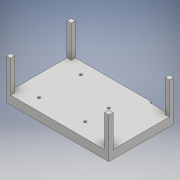
# Autodesk Inventor part: Back Plate test02
Saved by Autodesk Inventor 2018 (Build 220112000, 112)
## iProperties
Created: 2022-01-10
Part Number: Back Plate test02
Material: Generic
Document SubType Name: Modeling
Designer: Stewart Alexander
Density: 1 g/cm^3
Appearance: Default
Author: Stewart Alexander
Autodesk Inventor part; units mm, degrees
ref_plane "YZ Plane" through (0, 0, 0) normal (1, 0, 0) x (0, 1, 0)
ref_plane "XZ Plane" through (0, 0, 0) normal (0, 1, 0) x (-1, 0, 0)
ref_plane "XY Plane" through (0, 0, 0) normal (0, 0, 1) x (1, 0, 0)
sketch "Arduino Uno" plane through (0, 0, 0) normal (0, 0, 1) x (1, 0, 0)
  line L0 (0, 0) -> (68.6, 0)
  line L1 (68.6, 0) -> (68.6, 53.3)
  line L2 (68.6, 53.3) -> (0, 53.3)
  line L3 (0, 53.3) -> (0, 0)
  circle A0 centre (15.3, 50.7) radius 1.5
  circle A1 centre (14, 2.5) radius 1.5
  circle A2 centre (66.1, 5.1) radius 1.5
  line L4 (0, 53.3) -> (66.1, 53.3)
  circle A3 centre (66.1, 33) radius 1.5
  dimension "d6" = 68.6
  dimension "d7" = 53.3
  dimension "d34" = 3
  dimension "d36" = 3
  dimension "d38" = 2.5
  dimension "d39" = 3
  dimension "d40" = 14
  dimension "d41" = 1.3
  dimension "d42" = 66.1
  dimension "d43" = 3
  dimension "d44" = 5.1
  dimension "d45" = 27.9
  dimension "d50" = 2.6
  dimension "d51" = 2.5
  dimension "d52" = 2.5
  constraints: 10 end point, 4 centre point, 2 parallel, 1 horizontal, 1 perpendicular, 1 point on line
  measures "d6" distance of L2.end L1.end
  measures "d7" distance of L0.end L1.end
  measures "d34" diameter of A0
  measures "d36" diameter of A1
  measures "d38" distance from line of L0 A1.centre
  measures "d39" diameter of A2
  measures "d40" distance from line of L3 A1.centre
  measures "d41" horizontal distance of A1.centre A0.centre
  measures "d42" distance of L2.end L4.end
  measures "d43" diameter of A3
  measures "d44" distance from line of L0 A2.centre
  measures "d45" distance of A2.centre A3.centre
  measures "d50" distance from line of L2 A0.centre
  measures "d51" distance from line of L1 A3.centre
  measures "d52" distance from line of L1 A2.centre
sketch "Sketch2" plane through (0, 0, 0) normal (0, 0, 1) x (1, 0, 0)
  line L0 (-7.6751, -4.0855) -> (1.5398, -4.0855)
  line L1 (-10.3008, -11.8098) -> (-10.3008, 64.9422)
  line L2 (-10.3008, 64.9422) -> (110.9472, 64.9422)
  line L3 (110.9472, 64.9422) -> (110.9472, -11.8098)
  line L4 (110.9472, -11.8098) -> (-10.3008, -11.8098)
  circle A0 centre (15.3, 50.7) radius 1.5 projected
  point P0 (0, 0)
  dimension "d27" = 4.366
  dimension "d28" = 76.752
  dimension "d29" = 121.248
  constraints: 10 end point, 4 perpendicular, 1 horizontal
  measures "d27" distance of L0.end point (0, 0)
  measures "d28" distance of L1.start L1.end
  measures "d29" distance of L1.end L2.end
extrude "Back Plate" add sketch "Sketch2" against normal blind 10 contours L1 L2 L3 L4 | A0
extrude "Uno Mounting Holes" cut sketch "Arduino Uno" against normal blind 5 contours A0 | A1 | A2 | A3
sketch "Sketch3" plane through (0, 0, 0) normal (0, 0, 1) x (1, 0, 0)
  line L0 (110.9472, 64.9422) -> (105.9472, 64.9422)
  line L1 (105.9472, 64.9422) -> (105.9472, 59.9422)
  line L2 (105.9472, 59.9422) -> (110.9472, 59.9422)
  line L3 (110.9472, 59.9422) -> (110.9472, 64.9422)
  line L4 (110.9472, -11.8098) -> (-10.3008, -11.8098) projected
  line L5 (110.9472, -11.8098) -> (105.9472, -11.8098)
  line L6 (105.9472, -11.8098) -> (105.9472, -6.8098)
  line L7 (105.9472, -6.8098) -> (110.9472, -6.8098)
  line L8 (110.9472, -6.8098) -> (110.9472, -11.8098)
  line L9 (-10.3008, -11.8098) -> (-10.3008, 64.9422) projected
  line L10 (-10.3008, 64.9422) -> (-5.3008, 64.9422)
  line L11 (-5.3008, 64.9422) -> (-5.3008, 59.9422)
  line L12 (-5.3008, 59.9422) -> (-10.3008, 59.9422)
  line L13 (-10.3008, 59.9422) -> (-10.3008, 64.9422)
  line L14 (-10.3008, -11.8098) -> (-5.3008, -11.8098)
  line L15 (-5.3008, -11.8098) -> (-5.3008, -6.8098)
  line L16 (-5.3008, -6.8098) -> (-10.3008, -6.8098)
  line L17 (-10.3008, -6.8098) -> (-10.3008, -11.8098)
  point P0 (0, 0)
  dimension "d53" = 5
  dimension "d54" = 5
  dimension "d55" = 5
  dimension "d56" = 5
  dimension "d57" = 5
  dimension "d58" = 5
  dimension "d59" = 5
  dimension "d60" = 5
  constraints: 32 end point, 8 parallel, 4 horizontal, 4 perpendicular
  measures "d53" distance of L2.end L1.end
  measures "d54" distance of L0.end L1.end
  measures "d55" distance of L6.end L7.end
  measures "d56" distance of L7.end L4.start
  measures "d57" distance of L11.end L12.end
  measures "d58" distance of L10.end L11.end
  measures "d59" distance of L14.end L15.end
  measures "d60" distance of L15.end L16.end
extrude "Frame Pillars" add sketch "Sketch3" along normal blind 38
sketch "Sketch4" plane through (0, 0, 0) normal (0, 0, 1) x (1, 0, 0)
  line L0 (-5.3008, 64.9422) -> (105.9472, 64.9422) projected
  line L1 (105.9472, 64.9422) -> (84.9472, 64.9422)
  line L2 (84.9472, 64.9422) -> (84.9472, 63.0922)
  line L3 (84.9472, 63.0922) -> (105.9472, 63.0922)
  line L4 (105.9472, 63.0922) -> (105.9472, 64.9422)
  point P0 (0, 0)
  dimension "d63" = 21
  dimension "d64" = 1.85
  constraints: 8 end point, 2 parallel, 1 horizontal, 1 perpendicular
  measures "d63" distance of L3.end L2.end
  measures "d64" distance of L1.end L2.end
extrude "SD Channel" cut sketch "Sketch4" against normal through all
body "Solid1"
